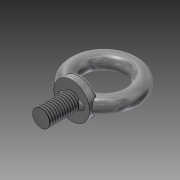
# Autodesk Inventor part: M12 EYE BOLT
Saved by Autodesk Inventor 2015 (Build 190159000, 159)
## iProperties
Created: 2015-04-21
Part Number: M12 EYE BOLT
Material: Steel, Carbon
Document SubType Name: Modeling
Designer: jacobus
Mass: 69.4163 g
Surface Area: 38.4404 cm^2
Volume: 8.84285 cm^3
Density: 7.85 g/cm^3
Appearance: Galvanized
Author: jacobus
Autodesk Inventor part; units mm, degrees
note: some values were not read from the file. Left out: dimensions or parameters whose unit could not be read.
ref_plane "YZ Plane" through (0, 0, 0) normal (1, 0, 0) x (0, 1, 0)
ref_plane "XZ Plane" through (0, 0, 0) normal (0, 1, 0) x (-1, 0, 0)
ref_plane "XY Plane" through (0, 0, 0) normal (0, 0, 1) x (1, 0, 0)
sketch "Sketch1" plane through (0, 0, 0) normal (1, 0, 0) x (0, 1, 0)
  line L0 (0, 16.3189) -> (0, -16.3189) construction
  line L1 (15.6465, 0) -> (-15.6465, 0) construction
  circle A0 centre (16, 0) radius 4.5
  line L2 (-19, 10.5) -> (-19, 0)
  circle A1 centre (-16, 0) radius 4.5 construction
  line L3 (-19, 10.5) -> (-15, 10.5)
  line L4 (-13, 8.5) -> (-13, 4.1533)
  arc A2 (-11.5, 0) -> (-12.5385, 2.8754) centre (-16, 0) ccw
  line L5 (-19, 0) -> (-11.5, 0)
  arc A3 (-13, 4.1533) -> (-12.5385, 2.8754) centre (-11, 4.1533) ccw
  arc A4 (-13, 8.5) -> (-15, 10.5) centre (-15, 8.5) ccw
  line L6 (-19, 0) -> (-37, 0)
  line L7 (-37, 0) -> (-37, 5)
  line L8 (-37, 5) -> (-19, 5)
  point P0 (0, 0)
  point P1 (0, 0)
  point P2 (-13, 10.5)
  point P3 (-13, 3.3541)
  dimension "D" = 9
  dimension "d1" = 16
  dimension "Emm" = 19
  dimension "B" = 21
  dimension "d4" = 6
  dimension "d5" = 2
  dimension "Amm" = 10
  dimension "Fmm" = 18
  constraints: 18 end point, 7 point on circle, 7 point on line, 4 centre point, 4 tangent, 3 horizontal, 3 perpendicular, 2 coincident, 2 midpoint, 2 vertical, 1 collinear, 1 equal radius, 1 symmetric about line, 4 other
  measures "D" diameter of A0
  measures "d1" distance from line of L0 A0.centre
  measures "Emm" distance between parallel lines of L0 L2
  measures "B" diameter of L2.start L1
  measures "d4" distance of L2.start point (-13, 10.5)
  measures "d5" radius of A3
  measures "Amm" diameter of L8 L1
  measures "Fmm" distance between parallel lines of L2 L7
revolve "Revolution1" add sketch "Sketch1" angle 360 about axis through (0, 0, 16.3189) along (0, 0, -1) contours A0
revolve "Revolution2" add sketch "Sketch1" angle 360 about axis through (0, -19, 0) along (0, -1, 0) contours L3 A4 L4 A3 A2 L5 L2 | L2 L6 L7 L8
thread "Thread7" size "M10x1.5" class "6g" standard "ANSI Metric M Profile" full length
equation "\"d1\" = 0.5 * Cmm + D"
equation "\"d4\" = 0.666667 * D"
equation "\"Cmm\" = 14"
body "Solid1"
